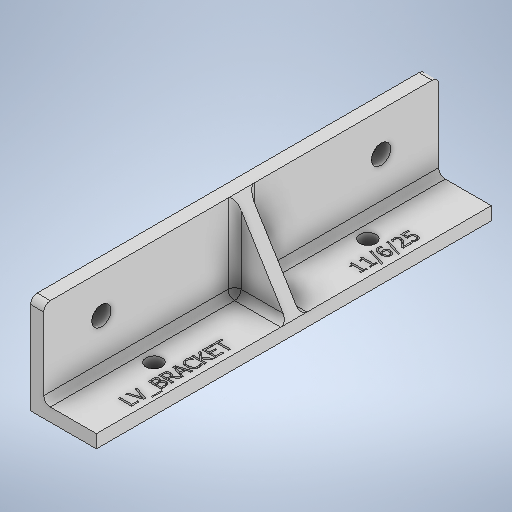
# Autodesk Inventor part: LV_Bracket_2
Saved by Autodesk Inventor 2025 (Build 290162000, 162)
## iProperties
Created: 2025-05-19
Part Number: LV_Bracket_2
Material: Generic
Document SubType Name: Modeling
Designer: mumin
Density: 1 g/cm^3
Appearance: Default
Author: mumin
Autodesk Inventor part; units mm, degrees
note: some values were not read from the file. Chosen so that the rebuilt part matches the saved one: direction of "LV Mount Hole"; direction of "80/20 Mount Hole".
ref_plane "YZ Plane" through (0, 0, 0) normal (1, 0, 0) x (0, 1, 0)
ref_plane "XZ Plane" through (0, 0, 0) normal (0, 1, 0) x (-1, 0, 0)
ref_plane "XY Plane" through (0, 0, 0) normal (0, 0, 1) x (1, 0, 0)
sketch "Sketch1" plane through (0, 0, 0) normal (0, 0, 1) x (1, 0, 0)
  line L0 (-4, 26) -> (-4, -4)
  line L1 (-4, -4) -> (16, -4)
  line L2 (16, -4) -> (16, 0)
  line L3 (16, 0) -> (0, 0)
  line L4 (0, 0) -> (0, 26)
  line L5 (0, 26) -> (-4, 26)
  point P0 (0, 0)
  dimension "d0" = 30
  dimension "d1" = 20
  dimension "d2" = 4
  dimension "d3" = 4
  constraints: 12 end point, 5 perpendicular, 1 vertical
  measures "d0" distance of L0.start L0.end
  measures "d1" distance of L0.end L1.end
  measures "d2" distance of L1.end L2.end
  measures "d3" distance between parallel lines of L4 L0
extrude "Base" add sketch "Sketch1" along normal mid plane 120
sketch "Sketch2" plane through (0, 0, 0) normal (0, 0, 1) x (1, 0, 0)
  line L0 (0, 0) -> (0, 26) projected
  line L1 (16, -4) -> (16, 0) projected
  line L2 (0, 26) -> (16, 0)
  line L3 (16, 0) -> (0, 0)
  constraints: 4 end point, 1 perpendicular
extrude "Center Truss" add sketch "Sketch2" along normal mid plane 4
fillet "Fillet1" radius 2 8 edges at (0, 0, 31) (0, 0, -31) (0, 13, 2) (8, 0, 2) (0, 13, -2) (8, 0, -2) (-2, 26, 60) (-2, 26, -60)
sketch "Sketch3" plane through (0, 2, 4) normal (1, 0, 0) x (0, 0, -1)
  line L0 (64, -6) -> (-56, -6) projected
  line L1 (8, 24) -> (0, 24) projected
  point P0 (4, -2)
  point P1 (-38.5, 12.28)
  point P2 (4, 24)
  dimension "d19" = 18.28
  dimension "d20" = 42.5
  constraints: 1 midpoint
  measures "d19" distance from line of L0 point (-38.5, 12.28)
  measures "d20" horizontal distance of point (4, 24) point (-38.5, 12.28)
hole "LV Mount Hole" at (0, 14.28, 42.5) direction (-1, 0, 0) diameter 5.9 depth 4
mirror "Mirror1" about plane through (0, 0, 0) normal (0, 0, 1) of "LV Mount Hole"
sketch "Sketch4" plane through (2, 0, 4) normal (0, 1, 0) x (1, 0, 0)
  line L0 (14, 0) -> (14, -56) projected
  line L1 (14, 8) -> (14, 0) projected
  point P0 (-2, 4)
  point P1 (4, -28.5)
  point P2 (14, -50)
  point P3 (14, 4)
  dimension "d28" = 10
  dimension "d29" = 32.5
  constraints: 1 midpoint
  measures "d28" distance from line of L0 point (4, -28.5)
  measures "d29" vertical distance of point (14, 4) point (4, -28.5)
hole "80/20 Mount Hole" at (6, 0, 32.5) direction (0, -1, 0) diameter 4.9 depth 4
mirror "Mirror2" about plane through (0, 0, 0) normal (0, 0, 1) of "80/20 Mount Hole"
sketch "Sketch5" plane through (-4, -4, -60) normal (-1, 0, 0) x (0, 0, 1)
  circle A0 centre (89, 18.28) radius 1.85
  line L0 (120, 28) -> (120, 0) projected
  circle A1 centre (29.5, 18.28) radius 1.85
  circle A2 centre (17.5, 18.28) radius 2.95 projected
  point P0 (60, 4)
  dimension "d31" = 3.7
  dimension "d32" = 31
  dimension "d33" = 3.7
  dimension "d34" = 12
  constraints: 2 centre point
  measures "d31" diameter of A0
  measures "d32" distance from line of L0 A0.centre
  measures "d33" diameter of A1
  measures "d34" distance of A1.centre A2.centre
extrude "Alignment Pins" add sketch "Sketch5" along normal blind 3 contours A0 | A1
fillet "Fillet2" radius 1 2 edges at (-7, 14.28, -32.35) (-7, 14.28, 27.15)
sketch "Sketch6" plane through (2, 0, 60) normal (0, 1, 0) x (1, 0, 0)
  line L0 (8.0338, 12.1618) -> (8.0338, 40.977) construction
  line L1 (8.0338, 40.977) -> (11.7586, 40.977) construction
  line L2 (11.7586, 40.977) -> (11.7586, 12.1618) construction
  line L3 (11.7586, 12.1618) -> (8.0338, 12.1618) construction
  line L4 (7.6408, 81.9717) -> (7.6408, 104.1889) construction
  line L5 (7.6408, 104.1889) -> (12.6878, 104.1889) construction
  line L6 (12.6878, 104.1889) -> (12.6878, 81.9717) construction
  line L7 (12.6878, 81.9717) -> (7.6408, 81.9717) construction
  line L8 (12.1051, 14.8847) -> (12.1051, 12.567)
  line L9 (12.1051, 12.567) -> (8.1051, 12.567)
  line L10 (8.1051, 12.567) -> (8.1051, 13.0986)
  line L11 (8.1051, 13.0986) -> (11.6318, 13.0986)
  line L12 (11.6318, 13.0986) -> (11.6318, 14.8847)
  line L13 (11.6318, 14.8847) -> (12.1051, 14.8847)
  line L14 (8.1051, 18.204) -> (12.1051, 16.8263)
  line L15 (12.1051, 16.8263) -> (12.1051, 16.2526)
  line L16 (12.1051, 16.2526) -> (8.1051, 14.8749)
  line L17 (8.1051, 14.8749) -> (8.1051, 15.4454)
  line L18 (8.1051, 15.4454) -> (11.4276, 16.554)
  line L19 (11.4276, 16.554) -> (8.1051, 17.6626)
  line L20 (8.1051, 17.6626) -> (8.1051, 18.204)
  line L21 (12.909, 21.225) -> (12.909, 18.1391)
  line L22 (12.909, 18.1391) -> (12.5622, 18.1391)
  line L23 (12.5622, 18.1391) -> (12.5622, 21.225)
  line L24 (12.5622, 21.225) -> (12.909, 21.225)
  spline S0 degree 2 poles (10.8766, 24.3012) (11.1748, 24.3012) (11.6318, 24.0743) (11.781, 23.8863) knots 0 0 0 1 2 2 2
  spline S1 degree 2 poles (11.781, 23.8863) (11.956, 23.6594) (12.1051, 23.144) (12.1051, 22.7356) knots 0 0 0 1 2 2 2
  line L25 (12.1051, 22.7356) -> (12.1051, 21.5881)
  line L26 (12.1051, 21.5881) -> (8.1051, 21.5881)
  line L27 (8.1051, 21.5881) -> (8.1051, 22.648)
  spline S2 degree 2 poles (8.1051, 22.648) (8.1051, 23.0759) (8.1602, 23.5038) (8.2672, 23.6983) knots 0 0 0 1 2 2 2
  spline S3 degree 2 poles (8.2672, 23.6983) (8.3806, 23.9155) (8.7534, 24.1132) (9.0062, 24.1132) knots 0 0 0 1 2 2 2
  spline S4 degree 2 poles (9.0062, 24.1132) (9.2882, 24.1132) (9.7356, 23.815) (9.862, 23.5524) knots 0 0 0 1 2 2 2
  line L28 (9.862, 23.5524) -> (9.8814, 23.5524)
  spline S5 degree 2 poles (9.8814, 23.5524) (9.9787, 23.909) (10.4941, 24.3012) (10.8766, 24.3012) knots 0 0 0 1 2 2 2
  spline S6 degree 2 poles (10.8993, 23.7469) (10.6724, 23.7469) (10.3806, 23.6172) (10.2769, 23.4228) knots 0 0 0 1 2 2 2
  spline S7 degree 2 poles (10.2769, 23.4228) (10.2121, 23.2963) (10.1732, 22.9981) (10.1732, 22.7226) knots 0 0 0 1 2 2 2
  line L29 (10.1732, 22.7226) -> (10.1732, 22.1197)
  line L30 (10.1732, 22.1197) -> (11.6513, 22.1197)
  line L31 (11.6513, 22.1197) -> (11.6513, 22.5508)
  spline S8 degree 2 poles (11.6513, 22.5508) (11.6513, 22.9009) (11.5865, 23.3028) (11.4827, 23.4584) knots 0 0 0 1 2 2 2
  spline S9 degree 2 poles (11.4827, 23.4584) (11.3758, 23.6075) (11.11, 23.7469) (10.8993, 23.7469) knots 0 0 0 1 2 2 2
  spline S10 degree 2 poles (9.0808, 23.5589) (8.9382, 23.5589) (8.7242, 23.4617) (8.6626, 23.3547) knots 0 0 0 1 2 2 2
  spline S11 degree 2 poles (8.6626, 23.3547) (8.5913, 23.225) (8.5589, 22.9106) (8.5589, 22.6286) knots 0 0 0 1 2 2 2
  line L32 (8.5589, 22.6286) -> (8.5589, 22.1197)
  line L33 (8.5589, 22.1197) -> (9.7291, 22.1197)
  line L34 (9.7291, 22.1197) -> (9.7291, 22.7226)
  spline S12 degree 2 poles (9.7291, 22.7226) (9.7291, 22.9722) (9.6772, 23.2088) (9.5962, 23.3352) knots 0 0 0 1 2 2 2
  spline S13 degree 2 poles (9.5962, 23.3352) (9.5184, 23.4584) (9.2688, 23.5589) (9.0808, 23.5589) knots 0 0 0 1 2 2 2
  line L35 (12.1051, 27.9252) -> (12.1051, 27.2347)
  line L36 (12.1051, 27.2347) -> (10.5135, 25.9706)
  line L37 (10.5135, 25.9706) -> (10.5135, 25.3612)
  line L38 (10.5135, 25.3612) -> (12.1051, 25.3612)
  line L39 (12.1051, 25.3612) -> (12.1051, 24.8296)
  line L40 (12.1051, 24.8296) -> (8.1051, 24.8296)
  line L41 (8.1051, 24.8296) -> (8.1051, 25.8604)
  spline S14 degree 2 poles (8.1051, 25.8604) (8.1051, 26.204) (8.1797, 26.6675) (8.3158, 26.8782) knots 0 0 0 1 2 2 2
  spline S15 degree 2 poles (8.3158, 26.8782) (8.4519, 27.0889) (8.8766, 27.332) (9.191, 27.332) knots 0 0 0 1 2 2 2
  spline S16 degree 2 poles (9.191, 27.332) (9.6286, 27.332) (10.2218, 26.8847) (10.3644, 26.5022) knots 0 0 0 1 2 2 2
  line L42 (10.3644, 26.5022) -> (12.1051, 27.9252)
  spline S17 degree 2 poles (9.2331, 26.7777) (9.0581, 26.7777) (8.7891, 26.6545) (8.7015, 26.5249) knots 0 0 0 1 2 2 2
  spline S18 degree 2 poles (8.7015, 26.5249) (8.627, 26.4114) (8.5654, 26.11) (8.5654, 25.8895) knots 0 0 0 1 2 2 2
  line L43 (8.5654, 25.8895) -> (8.5654, 25.3612)
  line L44 (8.5654, 25.3612) -> (10.0694, 25.3612)
  line L45 (10.0694, 25.3612) -> (10.0694, 25.8279)
  spline S19 degree 2 poles (10.0694, 25.8279) (10.0694, 26.0581) (9.9884, 26.4244) (9.862, 26.5508) knots 0 0 0 1 2 2 2
  spline S20 degree 2 poles (9.862, 26.5508) (9.7518, 26.6675) (9.4406, 26.7777) (9.2331, 26.7777) knots 0 0 0 1 2 2 2
  line L46 (12.1051, 27.8117) -> (8.1051, 29.1602)
  line L47 (8.1051, 29.1602) -> (8.1051, 29.815)
  line L48 (8.1051, 29.815) -> (12.1051, 31.1634)
  line L49 (12.1051, 31.1634) -> (12.1051, 30.6027)
  line L50 (12.1051, 30.6027) -> (10.9868, 30.2396)
  line L51 (10.9868, 30.2396) -> (10.9868, 28.7129)
  line L52 (10.9868, 28.7129) -> (12.1051, 28.3498)
  line L53 (12.1051, 28.3498) -> (12.1051, 27.8117)
  line L54 (10.533, 30.0937) -> (8.6497, 29.4746)
  line L55 (8.6497, 29.4746) -> (10.533, 28.8587)
  line L56 (10.533, 28.8587) -> (10.533, 30.0937)
  spline S21 degree 2 poles (12.1764, 33.1051) (12.1764, 32.7161) (11.9139, 32.0581) (11.6513, 31.8182) knots 0 0 0 1 2 2 2
  spline S22 degree 2 poles (11.6513, 31.8182) (11.392, 31.5783) (10.614, 31.3158) (10.1083, 31.3158) knots 0 0 0 1 2 2 2
  spline S23 degree 2 poles (10.1083, 31.3158) (9.6059, 31.3158) (8.8604, 31.5719) (8.5848, 31.815) knots 0 0 0 1 2 2 2
  spline S24 degree 2 poles (8.5848, 31.815) (8.3158, 32.0548) (8.0338, 32.7096) (8.0338, 33.1148) knots 0 0 0 1 2 2 2
  spline S25 degree 2 poles (8.0338, 33.1148) (8.0338, 33.3158) (8.0921, 33.6691) (8.1375, 33.8182) knots 0 0 0 1 2 2 2
  spline S26 degree 2 poles (8.1375, 33.8182) (8.1797, 33.9479) (8.2996, 34.2169) (8.3709, 34.3498) knots 0 0 0 1 2 2 2
  line L57 (8.3709, 34.3498) -> (9.0127, 34.3498)
  line L58 (9.0127, 34.3498) -> (9.0127, 34.3077)
  spline S27 degree 2 poles (9.0127, 34.3077) (8.9479, 34.2364) (8.7664, 34.0159) (8.6788, 33.8571) knots 0 0 0 1 2 2 2
  spline S28 degree 2 poles (8.6788, 33.8571) (8.5946, 33.7048) (8.4876, 33.345) (8.4876, 33.1116) knots 0 0 0 1 2 2 2
  spline S29 degree 2 poles (8.4876, 33.1116) (8.4876, 32.8555) (8.6983, 32.3984) (8.8993, 32.2266) knots 0 0 0 1 2 2 2
  spline S30 degree 2 poles (8.8993, 32.2266) (9.1035, 32.0581) (9.7226, 31.8701) (10.1083, 31.8701) knots 0 0 0 1 2 2 2
  spline S31 degree 2 poles (10.1083, 31.8701) (10.52, 31.8701) (11.1132, 32.0678) (11.3174, 32.2396) knots 0 0 0 1 2 2 2
  spline S32 degree 2 poles (11.3174, 32.2396) (11.5152, 32.4082) (11.7161, 32.8587) (11.7161, 33.1116) knots 0 0 0 1 2 2 2
  spline S33 degree 2 poles (11.7161, 33.1116) (11.7161, 33.3417) (11.6027, 33.7339) (11.5184, 33.8863) knots 0 0 0 1 2 2 2
  spline S34 degree 2 poles (11.5184, 33.8863) (11.4341, 34.0322) (11.2591, 34.2493) (11.1975, 34.3109) knots 0 0 0 1 2 2 2
  line L59 (11.1975, 34.3109) -> (11.1975, 34.3498)
  line L60 (11.1975, 34.3498) -> (11.8328, 34.3498)
  spline S35 degree 2 poles (11.8328, 34.3498) (11.8944, 34.2169) (12.0079, 33.9835) (12.0597, 33.8182) knots 0 0 0 1 2 2 2
  spline S36 degree 2 poles (12.0597, 33.8182) (12.1181, 33.6432) (12.1764, 33.345) (12.1764, 33.1051) knots 0 0 0 1 2 2 2
  line L61 (12.1051, 37.7631) -> (12.1051, 37.0727)
  line L62 (12.1051, 37.0727) -> (10.2445, 35.6108)
  line L63 (10.2445, 35.6108) -> (10.507, 35.3774)
  line L64 (10.507, 35.3774) -> (12.1051, 35.3774)
  line L65 (12.1051, 35.3774) -> (12.1051, 34.8458)
  line L66 (12.1051, 34.8458) -> (8.1051, 34.8458)
  line L67 (8.1051, 34.8458) -> (8.1051, 35.3774)
  line L68 (8.1051, 35.3774) -> (9.943, 35.3774)
  line L69 (9.943, 35.3774) -> (8.1051, 37.0176)
  line L70 (8.1051, 37.0176) -> (8.1051, 37.6659)
  line L71 (8.1051, 37.6659) -> (9.8912, 36.0095)
  line L72 (9.8912, 36.0095) -> (12.1051, 37.7631)
  line L73 (12.1051, 38.0808) -> (8.1051, 38.0808)
  line L74 (8.1051, 38.0808) -> (8.1051, 40.5832)
  line L75 (8.1051, 40.5832) -> (8.5784, 40.5832)
  line L76 (8.5784, 40.5832) -> (8.5784, 38.6124)
  line L77 (8.5784, 38.6124) -> (9.674, 38.6124)
  line L78 (9.674, 38.6124) -> (9.674, 40.4503)
  line L79 (9.674, 40.4503) -> (10.1472, 40.4503)
  line L80 (10.1472, 40.4503) -> (10.1472, 38.6124)
  line L81 (10.1472, 38.6124) -> (11.6318, 38.6124)
  line L82 (11.6318, 38.6124) -> (11.6318, 40.5832)
  line L83 (11.6318, 40.5832) -> (12.1051, 40.5832)
  line L84 (12.1051, 40.5832) -> (12.1051, 38.0808)
  line L85 (12.1051, 42.1002) -> (8.5784, 42.1002)
  line L86 (8.5784, 42.1002) -> (8.5784, 40.7583)
  line L87 (8.5784, 40.7583) -> (8.1051, 40.7583)
  line L88 (8.1051, 40.7583) -> (8.1051, 43.9738)
  line L89 (8.1051, 43.9738) -> (8.5784, 43.9738)
  line L90 (8.5784, 43.9738) -> (8.5784, 42.6318)
  line L91 (8.5784, 42.6318) -> (12.1051, 42.6318)
  line L92 (12.1051, 42.6318) -> (12.1051, 42.1002)
  line L93 (11.8191, 84.5292) -> (11.8191, 82.5778)
  line L94 (11.8191, 82.5778) -> (11.4106, 82.5778)
  line L95 (11.4106, 82.5778) -> (11.4106, 83.3039)
  line L96 (11.4106, 83.3039) -> (8.7299, 83.3039)
  line L97 (8.7299, 83.3039) -> (8.7299, 82.5778)
  line L98 (8.7299, 82.5778) -> (8.3636, 82.5778)
  spline S37 degree 2 poles (8.3636, 82.5778) (8.3636, 82.9895) (8.1302, 83.3785) (7.8061, 83.4044) knots 0 0 0 1 2 2 2
  line L99 (7.8061, 83.4044) -> (7.8061, 83.8193)
  line L100 (7.8061, 83.8193) -> (11.4106, 83.8193)
  line L101 (11.4106, 83.8193) -> (11.4106, 84.5292)
  line L102 (11.4106, 84.5292) -> (11.8191, 84.5292)
  line L103 (11.8191, 87.5308) -> (11.8191, 85.5795)
  line L104 (11.8191, 85.5795) -> (11.4106, 85.5795)
  line L105 (11.4106, 85.5795) -> (11.4106, 86.3056)
  line L106 (11.4106, 86.3056) -> (8.7299, 86.3056)
  line L107 (8.7299, 86.3056) -> (8.7299, 85.5795)
  line L108 (8.7299, 85.5795) -> (8.3636, 85.5795)
  spline S38 degree 2 poles (8.3636, 85.5795) (8.3636, 85.9911) (8.1302, 86.3801) (7.8061, 86.406) knots 0 0 0 1 2 2 2
  line L109 (7.8061, 86.406) -> (7.8061, 86.821)
  line L110 (7.8061, 86.821) -> (11.4106, 86.821)
  line L111 (11.4106, 86.821) -> (11.4106, 87.5308)
  line L112 (11.4106, 87.5308) -> (11.8191, 87.5308)
  line L113 (7.6408, 89.9295) -> (12.6878, 88.3639)
  line L114 (12.6878, 88.3639) -> (12.6878, 87.9101)
  line L115 (12.6878, 87.9101) -> (7.6408, 89.4693)
  line L116 (7.6408, 89.4693) -> (7.6408, 89.9295)
  spline S39 degree 2 poles (10.5225, 92.8988) (10.8304, 92.8988) (11.3523, 92.6945) (11.5273, 92.5227) knots 0 0 0 1 2 2 2
  spline S40 degree 2 poles (11.5273, 92.5227) (11.7121, 92.3445) (11.9033, 91.8971) (11.9033, 91.6281) knots 0 0 0 1 2 2 2
  spline S41 degree 2 poles (11.9033, 91.6281) (11.9033, 91.359) (11.7218, 90.915) (11.5403, 90.7464) knots 0 0 0 1 2 2 2
  spline S42 degree 2 poles (11.5403, 90.7464) (11.3231, 90.5389) (10.5938, 90.3056) (10.0622, 90.3056) knots 0 0 0 1 2 2 2
  spline S43 degree 2 poles (10.0622, 90.3056) (9.5403, 90.3056) (8.7007, 90.5195) (8.3896, 90.7432) knots 0 0 0 1 2 2 2
  spline S44 degree 2 poles (8.3896, 90.7432) (8.0849, 90.9603) (7.7445, 91.6475) (7.7445, 92.0981) knots 0 0 0 1 2 2 2
  spline S45 degree 2 poles (7.7445, 92.0981) (7.7445, 92.231) (7.7704, 92.4644) (7.7996, 92.5519) knots 0 0 0 1 2 2 2
  line L117 (7.7996, 92.5519) -> (8.315, 92.5519)
  line L118 (8.315, 92.5519) -> (8.315, 92.5292)
  spline S46 degree 2 poles (8.315, 92.5292) (8.2761, 92.4547) (8.208, 92.1824) (8.208, 92.0268) knots 0 0 0 1 2 2 2
  spline S47 degree 2 poles (8.208, 92.0268) (8.208, 91.5276) (8.8823, 90.915) (9.5435, 90.8566) knots 0 0 0 1 2 2 2
  spline S48 degree 2 poles (9.5435, 90.8566) (9.4106, 91.0479) (9.2648, 91.4498) (9.2648, 91.6897) knots 0 0 0 1 2 2 2
  spline S49 degree 2 poles (9.2648, 91.6897) (9.2648, 91.9231) (9.3588, 92.2731) (9.5014, 92.4644) knots 0 0 0 1 2 2 2
  spline S50 degree 2 poles (9.5014, 92.4644) (9.6667, 92.6848) (10.1789, 92.8988) (10.5225, 92.8988) knots 0 0 0 1 2 2 2
  spline S51 degree 2 poles (10.5451, 92.3542) (10.2988, 92.3542) (9.9649, 92.2245) (9.8482, 92.0819) knots 0 0 0 1 2 2 2
  spline S52 degree 2 poles (9.8482, 92.0819) (9.7639, 91.9749) (9.7088, 91.7091) (9.7088, 91.5697) knots 0 0 0 1 2 2 2
  spline S53 degree 2 poles (9.7088, 91.5697) (9.7088, 91.3817) (9.8223, 91.0284) (9.9293, 90.8566) knots 0 0 0 1 2 2 2
  spline S54 degree 2 poles (9.9293, 90.8566) (9.9876, 90.8534) (10.0978, 90.8469) (10.1821, 90.8469) knots 0 0 0 1 2 2 2
  spline S55 degree 2 poles (10.1821, 90.8469) (10.597, 90.8469) (11.1059, 91.009) (11.2388, 91.1321) knots 0 0 0 1 2 2 2
  spline S56 degree 2 poles (11.2388, 91.1321) (11.3652, 91.2456) (11.4657, 91.4919) (11.4657, 91.6313) knots 0 0 0 1 2 2 2
  spline S57 degree 2 poles (11.4657, 91.6313) (11.4657, 91.9555) (11.0054, 92.3542) (10.5451, 92.3542) knots 0 0 0 1 2 2 2
  line L119 (7.6408, 95.0349) -> (12.6878, 93.4693)
  line L120 (12.6878, 93.4693) -> (12.6878, 93.0154)
  line L121 (12.6878, 93.0154) -> (7.6408, 94.5746)
  line L122 (7.6408, 94.5746) -> (7.6408, 95.0349)
  line L123 (11.8191, 97.9425) -> (11.8191, 95.4757)
  line L124 (11.8191, 95.4757) -> (11.2518, 95.4757)
  spline S58 degree 2 poles (11.2518, 95.4757) (11.0022, 95.7415) (10.5387, 96.2148) (10.2891, 96.4417) knots 0 0 0 1 2 2 2
  spline S59 degree 2 poles (10.2891, 96.4417) (9.7866, 96.8988) (9.1837, 97.2326) (8.8628, 97.2326) knots 0 0 0 1 2 2 2
  spline S60 degree 2 poles (8.8628, 97.2326) (8.6943, 97.2326) (8.4414, 97.1289) (8.3604, 97.0349) knots 0 0 0 1 2 2 2
  spline S61 degree 2 poles (8.3604, 97.0349) (8.2793, 96.9409) (8.1983, 96.6945) (8.1983, 96.5454) knots 0 0 0 1 2 2 2
  spline S62 degree 2 poles (8.1983, 96.5454) (8.1983, 96.4028) (8.2696, 96.1111) (8.3247, 95.9782) knots 0 0 0 1 2 2 2
  spline S63 degree 2 poles (8.3247, 95.9782) (8.3701, 95.8647) (8.4998, 95.654) (8.5451, 95.5892) knots 0 0 0 1 2 2 2
  line L125 (8.5451, 95.5892) -> (8.5451, 95.56)
  line L126 (8.5451, 95.56) -> (7.9746, 95.56)
  spline S64 degree 2 poles (7.9746, 95.56) (7.8936, 95.7253) (7.7348, 96.3185) (7.7348, 96.5843) knots 0 0 0 1 2 2 2
  spline S65 degree 2 poles (7.7348, 96.5843) (7.7348, 97.1451) (8.328, 97.7772) (8.8336, 97.7772) knots 0 0 0 1 2 2 2
  spline S66 degree 2 poles (8.8336, 97.7772) (9.0703, 97.7772) (9.4657, 97.667) (9.6343, 97.5697) knots 0 0 0 1 2 2 2
  spline S67 degree 2 poles (9.6343, 97.5697) (9.8093, 97.4725) (10.1529, 97.1905) (10.3182, 97.0349) knots 0 0 0 1 2 2 2
  spline S68 degree 2 poles (10.3182, 97.0349) (10.5938, 96.7821) (11.1837, 96.1629) (11.3555, 95.9782) knots 0 0 0 1 2 2 2
  line L127 (11.3555, 95.9782) -> (11.3555, 97.9425)
  line L128 (11.3555, 97.9425) -> (11.8191, 97.9425)
  spline S69 degree 2 poles (10.5484, 100.902) (10.8369, 100.902) (11.3296, 100.7172) (11.5111, 100.5487) knots 0 0 0 1 2 2 2
  spline S70 degree 2 poles (11.5111, 100.5487) (11.6926, 100.3801) (11.9033, 99.8777) (11.9033, 99.5665) knots 0 0 0 1 2 2 2
  spline S71 degree 2 poles (11.9033, 99.5665) (11.9033, 99.2812) (11.7769, 98.7237) (11.6764, 98.5195) knots 0 0 0 1 2 2 2
  line L129 (11.6764, 98.5195) -> (11.1092, 98.5195)
  line L130 (11.1092, 98.5195) -> (11.1092, 98.5584)
  spline S72 degree 2 poles (11.1092, 98.5584) (11.1545, 98.62) (11.2712, 98.8501) (11.3231, 98.9895) knots 0 0 0 1 2 2 2
  spline S73 degree 2 poles (11.3231, 98.9895) (11.3782, 99.1483) (11.4398, 99.4109) (11.4398, 99.5762) knots 0 0 0 1 2 2 2
  spline S74 degree 2 poles (11.4398, 99.5762) (11.4398, 99.7383) (11.3231, 100.043) (11.1967, 100.1532) knots 0 0 0 1 2 2 2
  spline S75 degree 2 poles (11.1967, 100.1532) (11.0767, 100.2537) (10.7591, 100.3574) (10.5451, 100.3574) knots 0 0 0 1 2 2 2
  spline S76 degree 2 poles (10.5451, 100.3574) (10.3312, 100.3574) (10.0589, 100.2407) (9.9682, 100.1305) knots 0 0 0 1 2 2 2
  spline S77 degree 2 poles (9.9682, 100.1305) (9.8677, 100.0171) (9.7834, 99.68) (9.7834, 99.4757) knots 0 0 0 1 2 2 2
  spline S78 degree 2 poles (9.7834, 99.4757) (9.7834, 99.2553) (9.8515, 98.8177) (9.8806, 98.6848) knots 0 0 0 1 2 2 2
  line L131 (9.8806, 98.6848) -> (7.8191, 98.6848)
  line L132 (7.8191, 98.6848) -> (7.8191, 100.8793)
  line L133 (7.8191, 100.8793) -> (8.2891, 100.8793)
  line L134 (8.2891, 100.8793) -> (8.2891, 99.2002)
  line L135 (8.2891, 99.2002) -> (9.3555, 99.2002)
  spline S79 degree 2 poles (9.3555, 99.2002) (9.3426, 99.2975) (9.3328, 99.4855) (9.3328, 99.5633) knots 0 0 0 1 2 2 2
  spline S80 degree 2 poles (9.3328, 99.5633) (9.3328, 99.8712) (9.4333, 100.2958) (9.5824, 100.4903) knots 0 0 0 1 2 2 2
  spline S81 degree 2 poles (9.5824, 100.4903) (9.7315, 100.6881) (10.1853, 100.902) (10.5484, 100.902) knots 0 0 0 1 2 2 2
  point P0 (-2, 60)
  constraints: 4 other
emboss "LABEL" sketch "Sketch6" operation cut depth 1 direction (0, -1, 0)
body "Solid1"
